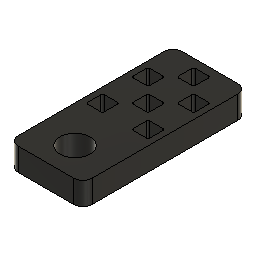
C-ChannelExtension (Autodesk Fusion 360 design; units mm, degrees)
Autodesk Fusion 360 part; units mm, degrees
sketch "Sketch1" plane through (0, 0, -6.0198) normal (0, 0, 1) x (-1, 0, 0)
  line L0 (-4.0409, -44.45) -> (3.9347, -44.45)
  line L1 (3.9347, -44.45) -> (3.9347, 6.35)
  line L2 (3.9347, 6.35) -> (-16.6393, 6.35)
  line L3 (-16.6393, 6.35) -> (-16.6393, -44.45)
  line L4 (-16.6393, -44.45) -> (-8.6637, -44.45)
  line L5 (-8.6637, -44.45) -> (-8.6637, -42.6466)
  arc A0 (-8.1557, -42.1386) -> (-8.6637, -42.6466) centre (-8.1557, -42.6466) ccw
  line L6 (-8.1557, -42.1386) -> (-4.5489, -42.1386)
  arc A1 (-4.0409, -42.6466) -> (-4.5489, -42.1386) centre (-4.5489, -42.6466) ccw
  line L7 (-4.0409, -42.6466) -> (-4.0409, -44.45)
  arc A2 (-8.1557, -29.4386) -> (-8.6637, -29.9466) centre (-8.1557, -29.9466) ccw
  line L8 (-8.1557, -29.4386) -> (-4.5489, -29.4386)
  arc A3 (-4.0409, -29.9466) -> (-4.5489, -29.4386) centre (-4.5489, -29.9466) ccw
  line L9 (-4.0409, -29.9466) -> (-4.0409, -33.5534)
  arc A4 (-4.5489, -34.0614) -> (-4.0409, -33.5534) centre (-4.5489, -33.5534) ccw
  line L10 (-4.5489, -34.0614) -> (-8.1557, -34.0614)
  arc A5 (-8.6637, -33.5534) -> (-8.1557, -34.0614) centre (-8.1557, -33.5534) ccw
  line L11 (-8.6637, -33.5534) -> (-8.6637, -29.9466)
  arc A6 (1.8011, -40.4114) -> (2.3091, -39.9034) centre (1.8011, -39.9034) ccw
  line L12 (1.8011, -40.4114) -> (-1.8057, -40.4114)
  arc A7 (-2.3137, -39.9034) -> (-1.8057, -40.4114) centre (-1.8057, -39.9034) ccw
  line L13 (-2.3137, -39.9034) -> (-2.3137, -36.2966)
  arc A8 (-1.8057, -35.7886) -> (-2.3137, -36.2966) centre (-1.8057, -36.2966) ccw
  line L14 (-1.8057, -35.7886) -> (1.8011, -35.7886)
  arc A9 (2.3091, -36.2966) -> (1.8011, -35.7886) centre (1.8011, -36.2966) ccw
  line L15 (2.3091, -36.2966) -> (2.3091, -39.9034)
  arc A10 (1.8011, -27.7114) -> (2.3091, -27.2034) centre (1.8011, -27.2034) ccw
  line L16 (1.8011, -27.7114) -> (-1.8057, -27.7114)
  arc A11 (-2.3137, -27.2034) -> (-1.8057, -27.7114) centre (-1.8057, -27.2034) ccw
  line L17 (-2.3137, -27.2034) -> (-2.3137, -23.5966)
  arc A12 (-1.8057, -23.0886) -> (-2.3137, -23.5966) centre (-1.8057, -23.5966) ccw
  line L18 (-1.8057, -23.0886) -> (1.8011, -23.0886)
  arc A13 (2.3091, -23.5966) -> (1.8011, -23.0886) centre (1.8011, -23.5966) ccw
  line L19 (2.3091, -23.5966) -> (2.3091, -27.2034)
  arc A14 (1.8011, -15.0114) -> (2.3091, -14.5034) centre (1.8011, -14.5034) ccw
  line L20 (1.8011, -15.0114) -> (-1.8057, -15.0114)
  arc A15 (-2.3137, -14.5034) -> (-1.8057, -15.0114) centre (-1.8057, -14.5034) ccw
  line L21 (-2.3137, -14.5034) -> (-2.3137, -10.8966)
  arc A16 (-1.8057, -10.3886) -> (-2.3137, -10.8966) centre (-1.8057, -10.8966) ccw
  line L22 (-1.8057, -10.3886) -> (1.8011, -10.3886)
  arc A17 (2.3091, -10.8966) -> (1.8011, -10.3886) centre (1.8011, -10.8966) ccw
  line L23 (2.3091, -10.8966) -> (2.3091, -14.5034)
  arc A18 (1.8011, -2.3114) -> (2.3091, -1.8034) centre (1.8011, -1.8034) ccw
  line L24 (1.8011, -2.3114) -> (-1.8057, -2.3114)
  arc A19 (-2.3137, -1.8034) -> (-1.8057, -2.3114) centre (-1.8057, -1.8034) ccw
  line L25 (-2.3137, -1.8034) -> (-2.3137, 1.8034)
  arc A20 (-1.8057, 2.3114) -> (-2.3137, 1.8034) centre (-1.8057, 1.8034) ccw
  line L26 (-1.8057, 2.3114) -> (1.8011, 2.3114)
  arc A21 (2.3091, 1.8034) -> (1.8011, 2.3114) centre (1.8011, 1.8034) ccw
  line L27 (2.3091, 1.8034) -> (2.3091, -1.8034)
  arc A22 (-10.8989, -40.4114) -> (-10.3909, -39.9034) centre (-10.8989, -39.9034) ccw
  line L28 (-10.8989, -40.4114) -> (-14.5057, -40.4114)
  arc A23 (-15.0137, -39.9034) -> (-14.5057, -40.4114) centre (-14.5057, -39.9034) ccw
  line L29 (-15.0137, -39.9034) -> (-15.0137, -36.2966)
  arc A24 (-14.5057, -35.7886) -> (-15.0137, -36.2966) centre (-14.5057, -36.2966) ccw
  line L30 (-14.5057, -35.7886) -> (-10.8989, -35.7886)
  arc A25 (-10.3909, -36.2966) -> (-10.8989, -35.7886) centre (-10.8989, -36.2966) ccw
  line L31 (-10.3909, -36.2966) -> (-10.3909, -39.9034)
  arc A26 (-10.8989, -27.7114) -> (-10.3909, -27.2034) centre (-10.8989, -27.2034) ccw
  line L32 (-10.8989, -27.7114) -> (-14.5057, -27.7114)
  arc A27 (-15.0137, -27.2034) -> (-14.5057, -27.7114) centre (-14.5057, -27.2034) ccw
  line L33 (-15.0137, -27.2034) -> (-15.0137, -23.5966)
  arc A28 (-14.5057, -23.0886) -> (-15.0137, -23.5966) centre (-14.5057, -23.5966) ccw
  line L34 (-14.5057, -23.0886) -> (-10.8989, -23.0886)
  arc A29 (-10.3909, -23.5966) -> (-10.8989, -23.0886) centre (-10.8989, -23.5966) ccw
  line L35 (-10.3909, -23.5966) -> (-10.3909, -27.2034)
  arc A30 (-10.8989, -15.0114) -> (-10.3909, -14.5034) centre (-10.8989, -14.5034) ccw
  line L36 (-10.8989, -15.0114) -> (-14.5057, -15.0114)
  arc A31 (-15.0137, -14.5034) -> (-14.5057, -15.0114) centre (-14.5057, -14.5034) ccw
  line L37 (-15.0137, -14.5034) -> (-15.0137, -10.8966)
  arc A32 (-14.5057, -10.3886) -> (-15.0137, -10.8966) centre (-14.5057, -10.8966) ccw
  line L38 (-14.5057, -10.3886) -> (-10.8989, -10.3886)
  arc A33 (-10.3909, -10.8966) -> (-10.8989, -10.3886) centre (-10.8989, -10.8966) ccw
  line L39 (-10.3909, -10.8966) -> (-10.3909, -14.5034)
  arc A34 (-10.8989, -2.3114) -> (-10.3909, -1.8034) centre (-10.8989, -1.8034) ccw
  line L40 (-10.8989, -2.3114) -> (-14.5057, -2.3114)
  arc A35 (-15.0137, -1.8034) -> (-14.5057, -2.3114) centre (-14.5057, -1.8034) ccw
  line L41 (-15.0137, -1.8034) -> (-15.0137, 1.8034)
  arc A36 (-14.5057, 2.3114) -> (-15.0137, 1.8034) centre (-14.5057, 1.8034) ccw
  line L42 (-14.5057, 2.3114) -> (-10.8989, 2.3114)
  arc A37 (-10.3909, 1.8034) -> (-10.8989, 2.3114) centre (-10.8989, 1.8034) ccw
  line L43 (-10.3909, 1.8034) -> (-10.3909, -1.8034)
  arc A38 (-8.6637, -8.1534) -> (-8.1557, -8.6614) centre (-8.1557, -8.1534) ccw
  line L44 (-8.6637, -8.1534) -> (-8.6637, -4.5466)
  arc A39 (-8.1557, -4.0386) -> (-8.6637, -4.5466) centre (-8.1557, -4.5466) ccw
  line L45 (-8.1557, -4.0386) -> (-4.5489, -4.0386)
  arc A40 (-4.0409, -4.5466) -> (-4.5489, -4.0386) centre (-4.5489, -4.5466) ccw
  line L46 (-4.0409, -4.5466) -> (-4.0409, -8.1534)
  arc A41 (-4.5489, -8.6614) -> (-4.0409, -8.1534) centre (-4.5489, -8.1534) ccw
  line L47 (-4.5489, -8.6614) -> (-8.1557, -8.6614)
  arc A42 (-8.1557, -16.7386) -> (-8.6637, -17.2466) centre (-8.1557, -17.2466) ccw
  line L48 (-8.1557, -16.7386) -> (-4.5489, -16.7386)
  arc A43 (-4.0409, -17.2466) -> (-4.5489, -16.7386) centre (-4.5489, -17.2466) ccw
  line L49 (-4.0409, -17.2466) -> (-4.0409, -20.8534)
  arc A44 (-4.5489, -21.3614) -> (-4.0409, -20.8534) centre (-4.5489, -20.8534) ccw
  line L50 (-4.5489, -21.3614) -> (-8.1557, -21.3614)
  arc A45 (-8.6637, -20.8534) -> (-8.1557, -21.3614) centre (-8.1557, -20.8534) ccw
  line L51 (-8.6637, -20.8534) -> (-8.6637, -17.2466)
  line L52 (1.3947, -23.5966) -> (-14.0993, -23.5966)
  line L53 (-16.6393, -21.0566) -> (-16.6393, 19.5834)
  line L54 (-14.0993, 22.1234) -> (1.3947, 22.1234)
  line L55 (3.9347, 19.5834) -> (3.9347, -21.0566)
  arc A46 (1.3947, -23.5966) -> (3.9347, -21.0566) centre (1.3947, -21.0566) ccw
  arc A47 (-16.6393, -21.0566) -> (-14.0993, -23.5966) centre (-14.0993, -21.0566) ccw
  arc A48 (-14.0993, 22.1234) -> (-16.6393, 19.5834) centre (-14.0993, 19.5834) ccw
  arc A49 (3.9347, 19.5834) -> (1.3947, 22.1234) centre (1.3947, 19.5834) ccw
  circle A50 centre (-6.3523, 14.0389) radius 4.191
  point P0 (3.9347, -23.5966)
  point P1 (-16.6393, -23.5966)
  point P2 (3.9347, 22.1234)
  dimension "d1" = 20.574
  dimension "d2" = 45.72
  dimension "d3" = 2.54
  dimension "d4" = 8.382
  constraint horizontal L52
  constraint vertical L53
  constraint horizontal L54
  constraint vertical L55
  constraint coincident L1 P0
  constraint coincident P0 L52
  constraint coincident P0 L55
  constraint tangent L52 A46
  constraint tangent L55 A46
  constraint coincident P1 L52
  constraint coincident P1 L53
  constraint tangent L52 A47
  constraint tangent L53 A47
  constraint equal A46 A47
  constraint tangent L53 A48
  constraint tangent L54 A48
  constraint equal A46 A48
  constraint coincident P2 L55
  constraint coincident P2 L54
  constraint tangent L55 A49
  constraint tangent L54 A49
  constraint equal A46 A49
  measures "d1" distance of P0 P1
  measures "d2" distance of P0 P2
  measures "d3" radius of A46
  measures "d4" diameter of A50
extrude "Extrude1" add sketch "Sketch1" along normal blind 6.35 contours L1 L2 L3 A12 L18 A13 A28 L34 A29 L52 L53 L55 A46 A47 | L2 L53 L54 L55 A48 A49 | A12 L18 A13 L52 A46 | A28 L34 A29 L52 A47
named bodies: "C-ChannelExtension"
